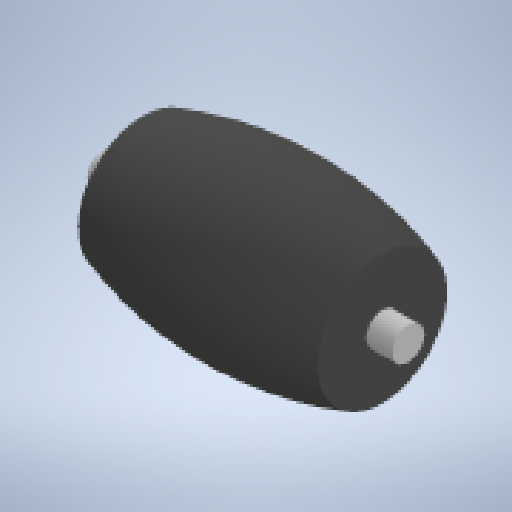
# Autodesk Inventor part: roller
Saved by Autodesk Inventor 2024.1 (Build 281209000, 209)
## iProperties
Created: 2024-11-26
Part Number: roller
Material: ゴム
Document SubType Name: Modeling
Designer: hibik
Density: 0.93 g/cm^3
Appearance: ゴム - 黒
Author: hibik
Autodesk Inventor part; units mm, degrees
ref_plane "YZ Plane" through (0, 0, 0) normal (1, 0, 0) x (0, 1, 0)
ref_plane "XZ Plane" through (0, 0, 0) normal (0, 1, 0) x (-1, 0, 0)
ref_plane "XY Plane" through (0, 0, 0) normal (0, 0, 1) x (1, 0, 0)
sketch "スケッチ1" plane through (0, 0, 0) normal (0, 0, 1) x (1, 0, 0)
  circle A0 centre (0, 0) radius 29
  line L0 (-9.25, 29) -> (9.25, 29)
  line L1 (9.25, 29) -> (9.25, 0)
  line L2 (9.25, 0) -> (-9.25, 0)
  line L3 (-9.25, 0) -> (-9.25, 29)
  line L4 (-9.25, 22.5) -> (9.25, 22.5)
  point P0 (9.25, 27.4852)
  point P1 (-9.25, 27.4852)
  dimension "d0" = 58
  dimension "d1" = 18.5
  dimension "d2" = 6.5
  constraints: 10 end point, 2 coincident, 2 parallel, 2 perpendicular, 2 point on line, 1 centre point, 1 horizontal, 1 midpoint, 1 tangent
  measures "d0" diameter of A0
  measures "d1" distance of L0.start L0.end
  measures "d2" distance between parallel lines of L0 L4
revolve "回転1" add sketch "スケッチ1" angle 360 about axis through (-9.25, 22.5, 0) along (1, 0, 0) contours L1 L4 L3 A0
sketch "スケッチ2" plane through (-9.25, 22.5, 0) normal (-1, 0, 0) x (0, 0, 1)
  circle A0 centre (0, 0) radius 1.25
  circle A1 centre (0, 0) radius 4.9852 projected
  point P0 (0, -22.5)
  dimension "d4" = 2.5
  constraints: 1 centre point, 1 concentric
  measures "d4" diameter of A0
extrude "押し出し1" add sketch "スケッチ2" along normal blind 3 contours A0
sketch "スケッチ3" plane through (9.25, 22.5, 0) normal (1, 0, 0) x (0, 0, -1)
  circle A0 centre (0, 0) radius 1.25 projected
  point P0 (0, -22.5)
extrude "押し出し2" add sketch "スケッチ3" along normal blind 3
